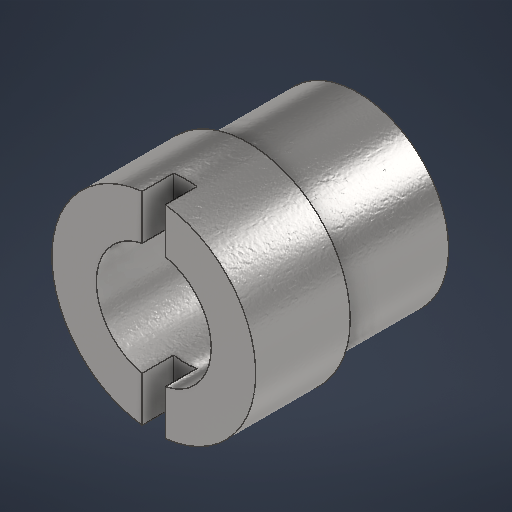
# Autodesk Inventor part: parça5
Saved by Autodesk Inventor 2025.4 (Build 294407000, 407)
## iProperties
Created: 2026-06-20
Part Number: parça5
Material: Generic
Document SubType Name: Modeling
Designer: yigithan
Density: 1 g/cm^3
Appearance: Galvanized
Author: yigithan
Autodesk Inventor part; units mm, degrees
ref_plane "YZ Plane" through (0, 0, 0) normal (1, 0, 0) x (0, 1, 0)
ref_plane "XZ Plane" through (0, 0, 0) normal (0, 1, 0) x (-1, 0, 0)
ref_plane "XY Plane" through (0, 0, 0) normal (0, 0, 1) x (1, 0, 0)
sketch "Sketch1" plane through (0, 0, 0) normal (0, 0, 1) x (1, 0, 0)
  circle A0 centre (0, 0) radius 9.12
  dimension "d0" = 18.24
  constraints: 1 centre point, 1 coincident
  measures "d0" diameter of A0
extrude "Extrusion1" add sketch "Sketch1" along normal blind 11.09
sketch "Sketch2" plane through (0, 0, 11.09) normal (0, 0, 1) x (1, 0, 0)
  circle A0 centre (0, 0) radius 10.285
  dimension "d3" = 20.57
  constraints: 1 centre point, 1 coincident
  measures "d3" diameter of A0
extrude "Extrusion2" add sketch "Sketch2" along normal blind 9.53
sketch "Sketch3" plane through (0, 0, 20.62) normal (0, 0, 1) x (1, 0, 0)
  circle A0 centre (0, 0) radius 5.795
  dimension "d6" = 11.59
  constraints: 1 centre point, 1 coincident
  measures "d6" diameter of A0
extrude "Extrusion3" cut sketch "Sketch3" against normal blind 33.78
sketch "Sketch4" plane through (0, 0, 0) normal (0, 1, 0) x (-1, 0, 0)
  line L0 (1.175, 17.44) -> (-1.175, 17.44)
  line L1 (-1.175, 17.44) -> (-1.175, 23.8)
  line L2 (-1.175, 23.8) -> (1.175, 23.8)
  line L3 (1.175, 23.8) -> (1.175, 17.44)
  line L4 (10.285, 20.62) -> (-10.285, 20.62) projected
  line L5 (1.175, 17.44) -> (-1.175, 23.8) construction
  line L6 (-1.175, 17.44) -> (1.175, 23.8) construction
  point P0 (0, 0)
  point P1 (0, 20.62)
  dimension "d9" = 2.35
  dimension "d10" = 6.36
  constraints: 12 end point, 3 midpoint, 2 parallel, 1 horizontal, 1 perpendicular
  measures "d9" distance of L1.end L2.end
  measures "d10" distance of L0.end L1.end
extrude "Extrusion4" cut sketch "Sketch4" along normal mid plane 33.78
body "Solid1"
